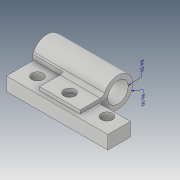
# Autodesk Inventor part: Cerniera 3
Saved by Autodesk Inventor 2019 (Build 230136000, 136)
## iProperties
Created: 2019-06-18
Part Number: Cerniera 3
Material: Generic
Document SubType Name: Modeling
Designer: giacomo
Density: 1 g/cm^3
Appearance: Default
Author: giacomo
Autodesk Inventor part; units mm, degrees
ref_plane "YZ Plane" through (0, 0, 0) normal (1, 0, 0) x (0, 1, 0)
ref_plane "XZ Plane" through (0, 0, 0) normal (0, 1, 0) x (-1, 0, 0)
ref_plane "XY Plane" through (0, 0, 0) normal (0, 0, 1) x (1, 0, 0)
sketch "Sketch1" plane through (0, 0, 0) normal (0, 1, 0) x (-1, 0, 0)
  line L0 (16.1753, 16.3636) -> (-28.8247, 16.3636)
  line L1 (-28.8247, 16.3636) -> (-28.8247, 6.3636)
  line L2 (16.1753, 6.3636) -> (16.1753, 16.3636)
  line L3 (-17.8247, 6.3636) -> (-17.8247, 1.3636)
  line L4 (-17.8247, 1.3636) -> (5.1753, 1.3636)
  line L5 (5.1753, 1.3636) -> (5.1753, 6.3636)
  line L6 (-28.8247, 6.3636) -> (-17.8247, 6.3636)
  line L7 (5.1753, 6.3636) -> (16.1753, 6.3636)
  point P0 (0, 0)
  dimension "d4" = 45
  dimension "d5" = 5
  dimension "d6" = 5
  dimension "d7" = 11
  dimension "d8" = 11
  dimension "d9" = 23
  dimension "d10" = 10
  constraints: 16 end point, 4 parallel, 1 horizontal, 1 perpendicular
  measures "d4" distance of L0.start L0.end
  measures "d5" distance of L4.end L5.end
  measures "d6" distance of L3.start L3.end
  measures "d7" distance of L1.end L3.start
  measures "d8" distance of L5.end L2.start
  measures "d9" distance of L3.end L4.end
  measures "d10" distance of L2.start L0.start
extrude "Extrusion1" add sketch "Sketch1" along normal blind 6
sketch "Sketch4" plane through (17.8247, 0, 6.3636) normal (1, 0, 0) x (0, 0, -1)
  circle A0 centre (8, 6.5) radius 6.5
  line L0 (0, 6) -> (5, 6) projected
  line L1 (0, 0) -> (0, 6) projected
  line L2 (0, 0) -> (5, 0) projected
  line L3 (5, 0) -> (16.9814, 0)
  point P0 (6.3636, 0)
  dimension "d20" = 13
  dimension "d36" = 8
  constraints: 2 end point, 1 centre point, 1 horizontal, 1 tangent
  measures "d20" diameter of A0
  measures "d36" distance from line of L1 A0.centre
extrude "Extrusion4" add sketch "Sketch4" against normal up to surface (23 mm away) contours A0
fillet "Fillet1" radius 12 2 edges at (6.3247, 0.7337, 1.3636) (6.3247, 0, 1.3636)
sketch "Sketch5" plane through (17.8247, 0, 6.3636) normal (1, 0, 0) x (0, 0, -1)
  circle A0 centre (8, 6.5) radius 6.5 projected
  circle A1 centre (8, 6.5) radius 2.5
  point P0 (6.3636, 0)
  point P1 (1.5193, 6)
  point P2 (7.416, 0.0263)
  dimension "d27" = 5
  constraints: 1 centre point, 1 coincident
  measures "d27" diameter of A1
extrude "Extrusion5" cut sketch "Sketch5" against normal through all contours A1
ref_plane "Work Plane1" through (17.8247, 6.5, -8.1364) normal (0, 0, 1) x (1, 0, 0)
sketch "Sketch6" plane through (0, 6, 0) normal (0, 1, 0) x (1, 0, 0)
  circle A0 centre (-9.0753, -9.6636) radius 2.5
  circle A1 centre (21.7247, -9.6636) radius 2.5
  line L0 (37.8247, 8.1364) -> (-25.1753, 8.1364) projected
  line L1 (28.8247, -16.3636) -> (28.8247, -6.3636) projected
  line L2 (-16.1753, -6.3636) -> (-16.1753, -16.3636) projected
  point P0 (0, 0)
  dimension "d33" = 5
  dimension "d34" = 5
  dimension "d35" = 17.8
  dimension "d37" = 17.8
  dimension "d38" = 7.1
  dimension "d39" = 30.8
  dimension "d40" = 7.1
  constraints: 2 centre point
  measures "d33" diameter of A0
  measures "d34" diameter of A1
  measures "d35" distance from line of L0 A1.centre
  measures "d37" distance from line of L0 A0.centre
  measures "d38" distance from line of L1 A1.centre
  measures "d39" distance of A0.centre A1.centre
  measures "d40" distance from line of L2 A0.centre
extrude "Extrusion6" cut sketch "Sketch6" against normal through all
move faces "Move1" translate (-2.5, 0, 0) faces at (17.8247, 2, 4.3758)
move faces "Move2" translate (2.5, 0, 0) faces at (-5.1753, 2, 4.3758) (8.4913, 6.099, -4.104)
sketch "Sketch7" plane through (0, 6, 0) normal (0, 1, 0) x (1, 0, 0)
  line L0 (-2.6753, -4.8444) -> (-2.6753, -6.3636) projected
  line L1 (-2.6753, -4.8444) -> (-2.6753, -14.145)
  line L2 (15.3247, -6.3636) -> (15.3247, -1.9193) projected
  line L3 (15.3247, -4.1415) -> (-2.6753, -4.1415)
  line L4 (-2.6753, -4.1415) -> (-2.6753, -15.1415)
  line L5 (-2.6753, -15.1415) -> (15.3247, -15.1415)
  line L6 (15.3247, -15.1415) -> (15.3247, -4.1415)
  point P0 (0, 0)
  dimension "d52" = 18
  dimension "d53" = 11
  constraints: 10 end point, 2 parallel, 1 collinear, 1 horizontal, 1 midpoint, 1 perpendicular
  measures "d52" distance of L4.end L5.end
  measures "d53" distance of L5.end L3.start
extrude "Extrusion7" add sketch "Sketch7" along normal blind 2
fillet "Fillet2" radius 2 1 edges at (6.3247, 8, 4.6882)
ref_plane "Work Plane5" through (0, 6, 0) normal (0, 1, 0) x (1, 0, 0)
sketch "Sketch8" plane through (0, 6, 0) normal (0, 1, 0) x (1, 0, 0)
  line L0 (-2.6753, -0.8636) -> (-2.6753, 4.1364) projected
  line L1 (-2.6753, -15.1415) -> (15.3247, -15.1415) projected
  line L2 (-2.6753, 0) -> (15.3247, 0)
  line L3 (15.3247, 0) -> (15.3247, -15.1415)
  line L4 (15.3247, -15.1415) -> (-2.6753, -15.1415)
  line L5 (-2.6753, -15.1415) -> (-2.6753, 0)
  point P0 (0, 0)
  constraints: 8 end point, 2 parallel, 1 horizontal, 1 perpendicular, 1 point on line
extrude "Extrusion8" cut sketch "Sketch8" along normal blind 0.5
ref_plane "Work Plane6" through (-2.6753, 0, 1.9193) normal (-1, 0, 0) x (0, 0, 1)
sketch "Sketch10" plane through (-2.6753, 0, 1.9193) normal (-1, 0, 0) x (0, 0, 1)
  line L0 (-1.0557, 6.5) -> (13.2222, 6.5) projected
  line L1 (13.2222, 6.5) -> (13.2222, 8) projected
  line L2 (4.1903, 8) -> (13.2222, 8) projected
  arc A0 (2.3677, 9.1765) -> (-2.9717, 0.0263) centre (-3.5557, 6.5) ccw projected
  arc A1 (-0.9468, 0.0374) -> (-2.9717, 0.0263) centre (-1.8936, -11.9252) ccw projected
  arc A2 (-0.9468, 0.0374) -> (0, 0) centre (0, 12) ccw projected
  line L3 (0, 0) -> (4.4443, 0) projected
  line L4 (4.4443, 0) -> (4.4443, 6) projected
  line L5 (4.4443, 6) -> (-1.1062, 6) projected
  arc A3 (-1.0557, 6.5) -> (-1.1062, 6) centre (-3.5557, 6.5) ccw projected
  arc A4 (2.3677, 9.1765) -> (4.1903, 8) centre (4.1903, 10) ccw projected
  point P0 (-1.9193, 0)
extrude "Extrusion9" add sketch "Sketch10" along normal up to surface (13.5 mm away)
sketch "Sketch11" plane through (-2.6753, 0, 1.9193) normal (-1, 0, 0) x (0, 0, 1)
  line L0 (2.7662, 9.2202) -> (17.7662, 9.2202)
  line L1 (17.7662, 9.2202) -> (17.7662, 6.2202)
  line L2 (17.7662, 6.2202) -> (2.7662, 6.2202)
  line L3 (2.7662, 6.2202) -> (2.7662, 9.2202)
  point P0 (-1.9193, 0)
  point P1 (-3.5557, 6.5)
  dimension "d82" = 15
  dimension "d83" = 3
  constraints: 8 end point, 2 parallel, 1 horizontal, 1 perpendicular
  measures "d82" distance of L0.start L0.end
  measures "d83" distance of L0.end L1.end
sketch "Sketch12" plane through (15.3247, 0, 6.3636) normal (1, 0, 0) x (0, 0, -1)
  arc A0 (3.5, 6.5) -> (3.5, 6.5) centre (8, 6.5) ccw
  line L0 (3.5, 6.5) -> (3.5, 6.5)
  circle A1 centre (8, 6.5) radius 2.5
  circle A2 centre (8, 6.5) radius 4.5
  point P0 (6.3636, 0)
  dimension "d72" = 2
  constraints: 3 centre point, 2 end point, 2 point on circle, 1 coincident
  measures "d72" radial gap between concentric circles of A1 A2
sketch "Sketch13" plane through (0, 8, 0) normal (0, 1, 0) x (1, 0, 0)
  line L0 (15.3247, -6.4035) -> (-2.6753, -6.4035) projected
  line L1 (15.3247, -15.1415) -> (15.3247, -0.8636) projected
  line L2 (-2.6753, -14.1415) -> (-2.6753, -2.35) projected
  circle A0 centre (6.3247, -10.8459) radius 2.5
  point P0 (0, 0)
  point P1 (15.3247, -3.7322)
  dimension "d68" = 5
  constraints: 1 centre point
  measures "d68" diameter of A0
extrude "Extrusion12" cut sketch "Sketch13" against normal through all
extrude "Extrusion13" cut sketch "Sketch12" against normal through all
extrude "Extrusion15" cut sketch "Sketch11" along normal up to surface (13.5 mm away)
ref_plane "Work Plane7" through (0, 1.5, 0) normal (0, 1, 0) x (1, 0, 0)
sketch "Sketch14" plane through (0, 1.5, 0) normal (0, 1, 0) x (1, 0, 0)
  circle A0 centre (6.3247, -10.8459) radius 2.5 projected
  line L0 (10.0747, -8.6808) -> (10.0747, -13.0109)
  line L1 (10.0747, -13.0109) -> (6.3247, -15.176)
  line L2 (6.3247, -15.176) -> (2.5747, -13.0109)
  line L3 (2.5747, -13.0109) -> (2.5747, -8.6808)
  line L4 (2.5747, -8.6808) -> (6.3247, -6.5157)
  line L5 (6.3247, -6.5157) -> (10.0747, -8.6808)
  line L6 (15.3247, -15.1415) -> (15.3247, -6.1096) projected
  point P0 (0, 0)
  dimension "d89" = 7.5
  constraints: 12 end point, 1 coincident, 1 parallel, 13 other
  measures "d89" distance between parallel lines of L0 L3
extrude "Extrusion16" cut sketch "Sketch14" along normal blind 3.15
body "Solid1"
